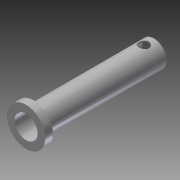
# Autodesk Inventor part: LongPin
Saved by Autodesk Inventor 2013 (Build 170138000, 138)
## iProperties
Created: 2014-05-23
Part Number: LongPin
Material: Steel
Document SubType Name: Modeling
Designer: nojessen
Density: 7.85 g/cm^3
Mass: 16.5266 g
Surface Area: 51.9232 cm^2
Volume: 2.1053 cm^3
Author: nojessen
Autodesk Inventor part; units mm, degrees
ref_plane "YZ Plane" through (0, 0, 0) normal (1, 0, 0) x (0, 1, 0)
ref_plane "XZ Plane" through (0, 0, 0) normal (0, 1, 0) x (-1, 0, 0)
sketch "Sketch1" plane through (0, 0, 0) normal (0, 0, 1) x (1, 0, 0)
  circle A0 centre (0, 0) radius 6.35
  circle A1 centre (0, 0) radius 5.715
  dimension "d0" = 12.7
  dimension "d1" = 11.43
  constraints: 2 centre point, 2 coincident
  measures "d0" diameter of A0
  measures "d1" diameter of A1
extrude "Extrusion1" add sketch "Sketch1" along normal blind 63.5
sketch "Sketch2" plane through (0, 0, 63.5) normal (0, 0, 1) x (1, 0, 0)
  circle A0 centre (0, 0) radius 6.35 projected
  circle A1 centre (0, 0) radius 9.525
  dimension "d4" = 19.05
  constraints: 1 centre point, 1 coincident
  measures "d4" diameter of A1
extrude "Extrusion2" add sketch "Sketch2" against normal blind 3.81
sketch "Sketch3" plane through (0, 0, 0) normal (0, 0, -1) x (-1, 0, 0)
  circle A0 centre (0, 0) radius 5.715 projected
  circle A1 centre (0, 0) radius 6.35 projected
  line L0 (0, 0) -> (-6.35, 0)
  constraints: 2 end point, 1 horizontal, 1 horizontal alignment, 1 other
ref_plane "Work Plane2" through (0, 6.35, 0) normal (0, 1, 0) x (1, 0, 0)
ref_plane "Work Plane1" through (0, 0, 0) normal (0, 1, 0) x (1, 0, 0)
sketch "Sketch4" plane through (0, 6.35, 0) normal (0, 1, 0) x (1, 0, 0)
  line L0 (0, 0) -> (0, -5.08)
  circle A0 centre (0, -5.08) radius 2.54
  dimension "d9" = 5.08
  dimension "d10" = 5.08
  constraints: 2 end point, 1 centre point, 1 coincident, 1 vertical
  measures "d9" distance of L0.start L0.end
  measures "d10" diameter of A0
extrude "Extrusion3" cut sketch "Sketch4" against normal blind 50.8
body "Solid1"
